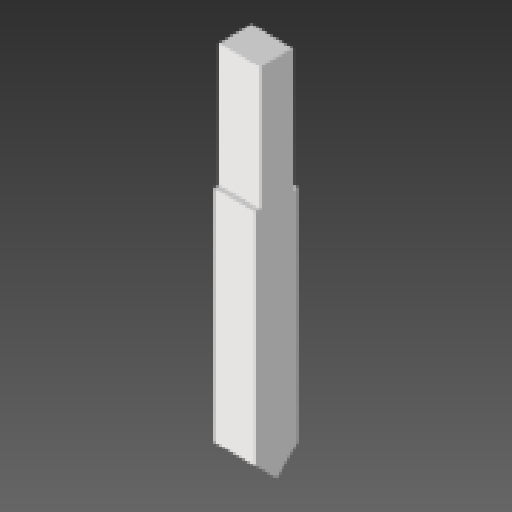
# Autodesk Inventor part: ForearmActuatorBodyBoundingBoxReal
Saved by Autodesk Inventor 2023 (Build 270158000, 158)
## iProperties
Created: 2023-03-25
Part Number: ForearmActuatorBodyBoundingBoxReal
Material: Generic
Document SubType Name: Modeling
Designer: Val
Density: 1 g/cm^3
Appearance: Default
Author: Val
Autodesk Inventor part; units mm, degrees
ref_plane "YZ Plane" through (0, 0, 0) normal (1, 0, 0) x (0, 1, 0)
ref_plane "XZ Plane" through (0, 0, 0) normal (0, 1, 0) x (-1, 0, 0)
ref_plane "XY Plane" through (0, 0, 0) normal (0, 0, 1) x (1, 0, 0)
sketch "Sketch1" plane through (0, 0, 0) normal (1, 0, 0) x (0, 1, 0)
  line L0 (0, 13) -> (134.5, 13)
  line L1 (134.5, 13) -> (134.5, -13)
  line L2 (134.5, -13) -> (0, -13)
  line L3 (0, -13) -> (0, 13) construction
  line L4 (134.5, 10) -> (209.702, 10)
  line L5 (209.702, 10) -> (209.702, -10)
  line L6 (209.702, -10) -> (134.5, -10)
  line L7 (134.5, -10) -> (134.5, 10)
  line L8 (209.702, -9) -> (209.702, 9) construction
  line L9 (134.5, 10) -> (208.702, 10) construction
  line L10 (134.5, 11.5) -> (134.5, -11.5) construction
  line L11 (133, 13) -> (0, 13) construction
  line L12 (133, -13) -> (8.0257, -13) construction
  line L13 (0, 13) -> (-13, 0)
  line L14 (-13, 0) -> (0, -13)
  line L15 (-57.5404, 0) -> (254.2424, 0) construction
  arc A0 (0, 13) -> (-8.5144, -9.8237) centre (0, 0) ccw construction
  point P0 (209.702, 0)
  constraints: 28 end point, 6 horizontal, 4 collinear, 4 parallel, 3 point on circle, 2 midpoint, 2 perpendicular, 2 point on line, 1 centre point, 10 other
extrude "Extrusion1" add sketch "Sketch1" along normal mid plane 26
body "Solid1"
